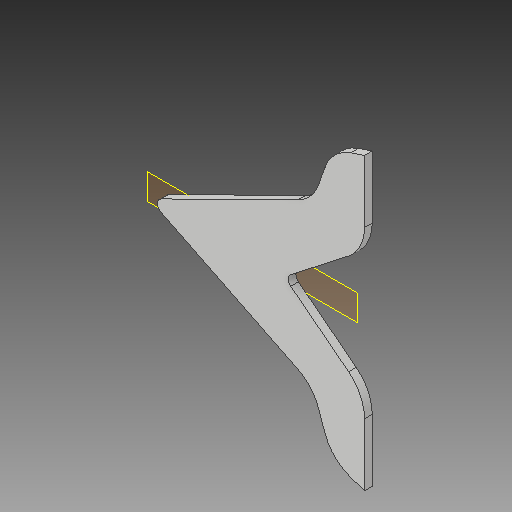
# Autodesk Inventor part: winglet
Saved by Autodesk Inventor 2017 (Build 210142000, 142)
## iProperties
Created: 2017-12-26
Part Number: winglet
Material: Generic
Document SubType Name: Modeling
Designer: will
Density: 1 g/cm^3
Appearance: Default
Author: will
Autodesk Inventor part; units mm, degrees
ref_plane "YZ Plane" through (0, 0, 0) normal (1, 0, 0) x (0, 1, 0)
ref_plane "XZ Plane" through (0, 0, 0) normal (0, 1, 0) x (-1, 0, 0)
ref_plane "XY Plane" through (0, 0, 0) normal (0, 0, 1) x (1, 0, 0)
ref_plane "Work Plane1" through (0, 0, 0) normal (0, 0, 1) x (1, 0, 0)
sketch "Sketch1" plane through (0, 0, 0) normal (0, 0, 1) x (1, 0, 0)
  line L0 (0, 0) -> (250.2323, 0)
  line L1 (0, 0) -> (214.0548, 105.6292)
  line L2 (214.0548, 105.6292) -> (238.5958, 175.5656)
  line L3 (238.5958, 175.5656) -> (281.6624, 190.0425)
  line L4 (281.6624, 190.0425) -> (281.6624, 81.9053)
  line L5 (281.6624, 81.9053) -> (176.6805, 0)
  constraints: 12 end point, 1 horizontal, 1 point on line, 1 vertical
extrude "Extrusion1" add sketch "Sketch1" along normal blind 10
mirror "Mirror1" about plane through (0, 0, 0) normal (0, -1, 0) of "Extrusion1"
fillet "Fillet1" radius 8.25 2 edges at (0, 0, 5) (176.6805, 0, 5)
fillet "Fillet2" radius 54.25 6 edges at (214.0548, 105.6292, 5) (238.5958, 175.5656, 5) (214.0548, -105.6292, 5) (238.5958, -175.5656, 5) (281.6624, 81.9053, 5) (281.6624, -81.9053, 5)
body "Solid1"
